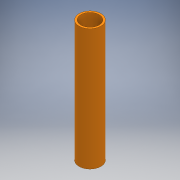
# Autodesk Inventor part: barra espaciadora
Saved by Autodesk Inventor 2018 (Build 220112000, 112)
## iProperties
Created: 2019-05-18
Part Number: barra espaciadora
Material: Generic
Document SubType Name: Modeling
Designer: JLVega003
Density: 1 g/cm^3
Appearance: Orange
Author: JLVega003
Autodesk Inventor part; units mm, degrees
ref_plane "YZ Plane" through (0, 0, 0) normal (1, 0, 0) x (0, 1, 0)
ref_plane "XZ Plane" through (0, 0, 0) normal (0, 1, 0) x (-1, 0, 0)
ref_plane "XY Plane" through (0, 0, 0) normal (0, 0, 1) x (1, 0, 0)
sketch "Sketch1" plane through (0, 0, 0) normal (0, 0, 1) x (1, 0, 0)
  circle A0 centre (0, 0) radius 19.05
  circle A1 centre (0, 0) radius 15.875
  dimension "d0" = 38.1
  dimension "d1" = 3.175
  constraints: 2 centre point, 2 coincident
  measures "d0" diameter of A0
  measures "d1" radial gap between concentric circles of A0 A1
extrude "Extrusion1" add sketch "Sketch1" along normal mid plane 212
body "Solid1"
